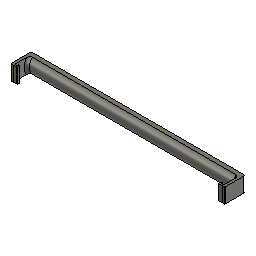
Test_rychka_90% (Autodesk Fusion 360 design; units mm, degrees)
Autodesk Fusion 360 part; units mm, degrees
note: some values were not read from the file. Set by a fixed rule: which sketch regions a step uses.
sketch "Sketch1" plane through (0, 0, 0) normal (0, 1, 0) x (1, 0, 0)
  line L0 (0, 0) -> (209.5, 0)
  line L1 (209.5, 0) -> (209.5, -39)
  line L2 (204.5, -8) -> (204.5, -36)
  line L3 (204.5, -40) -> (208.5, -40)
  line L4 (204.5, -40) -> (198, -40)
  line L5 (203.5, -37) -> (201, -37)
  line L6 (200, -36) -> (200, -35.5)
  line L7 (199, -34.5) -> (198, -34.5)
  line L8 (197, -35.5) -> (197, -39)
  arc A0 (200, -35.5) -> (199, -34.5) centre (199, -35.5) ccw
  arc A1 (198, -34.5) -> (197, -35.5) centre (198, -35.5) ccw
  arc A2 (200, -36) -> (201, -37) centre (201, -36) ccw
  arc A3 (203.5, -37) -> (204.5, -36) centre (203.5, -36) ccw
  arc A4 (197, -39) -> (198, -40) centre (198, -39) ccw
  arc A5 (208.5, -40) -> (209.5, -39) centre (208.5, -39) ccw
  line L9 (0, -8) -> (204.5, -8)
  line L10 (0, 0) -> (0, 20)
  arc A6 (-201, -37) -> (-200, -36) centre (-201, -36) ccw
  line L11 (-204.5, -8) -> (-204.5, -36)
  arc A7 (-199, -34.5) -> (-200, -35.5) centre (-199, -35.5) ccw
  line L12 (0, -8) -> (-204.5, -8)
  arc A8 (-198, -40) -> (-197, -39) centre (-198, -39) ccw
  line L13 (-200, -36) -> (-200, -35.5)
  line L14 (-204.5, -40) -> (-198, -40)
  line L15 (-204.5, -40) -> (-208.5, -40)
  line L16 (0, 0) -> (-209.5, 0)
  arc A9 (-204.5, -36) -> (-203.5, -37) centre (-203.5, -36) ccw
  line L17 (-203.5, -37) -> (-201, -37)
  line L18 (-199, -34.5) -> (-198, -34.5)
  line L19 (-209.5, 0) -> (-209.5, -39)
  line L20 (-197, -35.5) -> (-197, -39)
  arc A10 (-209.5, -39) -> (-208.5, -40) centre (-208.5, -39) ccw
  arc A11 (-197, -35.5) -> (-198, -34.5) centre (-198, -35.5) ccw
  point P0 (209.5, -40)
  point P1 (200, -37)
  point P2 (200, -34.5)
  point P3 (197, -34.5)
  point P4 (197, -40)
  point P5 (-209.5, -40)
  point P6 (-197, -40)
  point P7 (-200, -37)
  point P8 (-200, -34.5)
  point P9 (-197, -34.5)
  dimension "d15" = 40
  dimension "d16" = 7.5
  dimension "d17" = 5.5
  dimension "d18" = 3
  dimension "d20" = 2.5
  dimension "d21" = 1
  dimension "d22" = 1
  dimension "d23" = 1
  dimension "d24" = 1
  constraint coincident L0.start L10.start
  constraint horizontal L0
  constraint perpendicular L0 L1
  constraint perpendicular L0 L2
  constraint perpendicular L1 L3
  constraint perpendicular L2 L4
  constraint perpendicular L2 L5
  constraint perpendicular L5 L6
  constraint perpendicular L2 L7
  constraint perpendicular L7 L8
  constraint coincident P2 L6
  constraint coincident P2 L7
  constraint tangent L6 A0
  constraint tangent L7 A0
  constraint coincident P3 L7
  constraint coincident P3 L8
  constraint tangent L7 A1
  constraint tangent L8 A1
  constraint equal A0 A1
  constraint coincident P1 L5
  constraint coincident P1 L6
  constraint tangent L5 A2
  constraint tangent L6 A2
  constraint coincident L3.start L2
  constraint tangent L2 A3
  constraint tangent L5 A3
  constraint coincident P4 L8
  constraint coincident L4 P4
  constraint tangent L8 A4
  constraint tangent L4 A4
  constraint coincident P0 L1
  constraint coincident P0 L3
  constraint tangent L1 A5
  constraint tangent L3 A5
  constraint equal A4 A5
  constraint perpendicular L0 L10
  constraint symmetric L0.start L10 L16.start
  constraint symmetric L0.end L10 L16.end
  constraint symmetric P0 L10 P5
  constraint symmetric L3.start L10 L14.start
  constraint symmetric P1 L10 P7
  constraint symmetric P2 L10 P8
  constraint symmetric P3 L10 P9
  constraint symmetric P4 L10 P6
  constraint symmetric L6.end L10 A7.end
  constraint symmetric L7.start L10 A7.start
  constraint symmetric A0 L10 A7
  constraint symmetric L7.end L10 L18.end
  constraint symmetric L8.start L10 L20.start
  constraint symmetric A1 L10 A11
  constraint symmetric L5.end L10 A6.start
  constraint symmetric L6.start L10 A6.end
  constraint symmetric A2 L10 A6
  constraint symmetric L2.end L10 L11.end
  constraint symmetric L5.start L10 A9.end
  constraint symmetric A3 L10 A9
  constraint symmetric L8.end L10 A8.end
  constraint symmetric L4.end L10 A8.start
  constraint symmetric A4 L10 A8
  constraint symmetric L1.end L10 L19.end
  constraint symmetric L3.end L10 L15.end
  constraint symmetric A5 L10 A10
  constraint symmetric L9.start L10 L12.start
  constraint symmetric L2.start L10 L11.start
  measures "d15" distance of L0.end P0
  measures "d16" distance of L3.start P4
  measures "d17" distance of P3 P4
  measures "d18" distance of P2 P3
  measures "d20" distance of P1 P2
  measures "d21" radius of A0
  measures "d22" radius of A2
  measures "d23" radius of A3
  measures "d24" radius of A4
extrude "Extrude1" add sketch "Sketch1" along normal blind 29
sketch "Sketch2" plane through (204.5, 0, 0) normal (-1, 0, 0) x (0, 0, 1)
  line L0 (8, 0) -> (36, 0)
  line L1 (36, 0) -> (36, 29)
  line L2 (36, 29) -> (8, 29)
  line L3 (8, 29) -> (8, 0)
  line L4 (8, 29) -> (8, 0)
  arc A0 (8, 0) -> (8, 29) centre (-7.4757, 14.5) ccw
  constraint coincident L2.end L3.start
  constraint coincident L0.start L3.end
extrude "Extrude2" add sketch "Sketch2" along normal blind 409 contours L3 L4 A0
fillet "Fillet1" radius 5 2 edges at (-204.5, 14.5, 13.7316) (204.5, 14.5, 13.7316)
fillet "Fillet2" radius 3 2 edges at (-209.5, 14.5, 0) (209.5, 14.5, 0)
